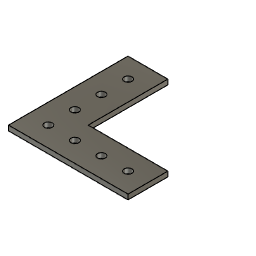
LBracket (Autodesk Fusion 360 design; units mm, degrees)
Autodesk Fusion 360 part; units mm, degrees
sketch "Sketch1" plane through (0, 0, 0) normal (0, 0, 1) x (1, 0, 0) in component "baseCorner"
  line L0 (0, 76.2) -> (0, 0)
  line L1 (0, 0) -> (76.2, 0)
  line L2 (76.2, 0) -> (76.2, 25.4)
  line L3 (76.2, 25.4) -> (25.4, 25.4)
  line L4 (25.4, 25.4) -> (25.4, 76.2)
  line L5 (25.4, 76.2) -> (0, 76.2)
  dimension "d12" = 25.4
  dimension "d13" = 25.4
  dimension "d14" = 76.2
  dimension "d15" = 76.2
  constraint vertical L0
  constraint perpendicular L0 L1
  constraint perpendicular L1 L2
  constraint perpendicular L2 L3
  constraint perpendicular L1 L4
  constraint perpendicular L0 L5
  constraint coincident L0.end L1.start
  measures "d12" distance of L0.start L4.end
  measures "d13" distance of L1.end L2.end
  measures "d14" distance of L0.end L1.end
  measures "d15" distance of L0.start L0.end
extrude "materialExtrude" add sketch "Sketch1" along normal blind 3.175 in component "baseCorner"
hole "initialHole" at (12.7, 12.7, 3.175) direction (0, 0, -1) diameter 4.9784 end through all in component "baseCorner"
pattern_linear "R-Pattern1" count 4 spacing 16.9333 along (1, 0, 0) count 4 spacing 16.9333 along (0, 1, 0) of "initialHole" in component "baseCorner"
component "baseCorner" placed x (1, 0, 0) y (0, 1, 0) z (0, 0, 1) at (0, 0, 0)
equation "thickness = 0.125 in"
equation "lengthX = 3 in"
equation "lengthY = 3 in"
equation "width = 1 in"
equation "holeD = 0.196 in" comment "#11 Rivet"
equation "numHolesX = 4"
equation "numHolesY = 4"
equation "d12 = width"
equation "d13 = width"
equation "d14 = lengthX"
equation "d15 = lengthY"
equation "d16 = thickness"
equation "d19 = holeD"
equation "d21 = width / 2"
equation "d22 = width / 2"
equation "d23 = numHolesX"
equation "d24 = numHolesY"
equation "d25 = ( lengthX - width ) / ( numHolesX - 1 )"
equation "d26 = ( lengthY - width ) / ( numHolesY - 1 )"
